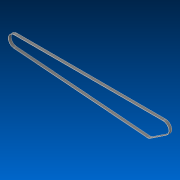
# Autodesk Inventor part: 225T x 9mm Wide Timing Belt (HTD 5mm)(217-3469)
Saved by Autodesk Inventor 2022 (Build 260153000, 153)
## iProperties
Created: 2022-01-07
Part Number: 225T x 9mm Wide Timing Belt (HTD 5mm)(217-3469)
Material: Fiberglass Batt
Document SubType Name: Modeling
Designer: omard
Density: 0.032 g/cm^3
Appearance: Gray
Author: omard
Autodesk Inventor part; units mm, degrees
ref_plane "YZ Plane" through (0, 0, 0) normal (1, 0, 0) x (0, 1, 0)
ref_plane "XZ Plane" through (0, 0, 0) normal (0, 1, 0) x (-1, 0, 0)
ref_plane "XY Plane" through (0, 0, 0) normal (0, 0, 1) x (1, 0, 0)
sketch "Sketch1" plane through (0, 0, 0) normal (0, 0, 1) x (1, 0, 0)
  arc A0 (0, 19.1008) -> (-1.5227, -19.04) centre (0, 0) ccw
  arc A1 (495.3, -19.1008) -> (505.9138, -15.8804) centre (495.3, 0) ccw construction
  line L0 (0, 19.1008) -> (495.3, 19.1008)
  line L1 (495.3, -19.1008) -> (0, -19.1008) construction
  line L2 (495.3, 20.1008) -> (0, 20.1008)
  arc A2 (0, 20.1008) -> (-1.6024, -20.0368) centre (0, 0) ccw
  line L3 (0, -20.1008) -> (495.3, -20.1008) construction
  arc A3 (495.3, -20.1008) -> (500.7083, -19.3595) centre (495.3, 0) ccw construction
  arc A4 (443.6141, -54.6381) -> (450.6749, -52.7999) centre (444.5, -43.561) ccw
  arc A5 (443.5344, -55.635) -> (451.2306, -53.6313) centre (444.5, -43.561) ccw
  line L4 (451.2306, -53.6313) -> (506.4695, -16.7118)
  line L5 (505.9138, -15.8804) -> (450.6749, -52.7999)
  line L6 (443.5344, -55.635) -> (-1.6024, -20.0368)
  line L7 (-1.5227, -19.04) -> (443.6141, -54.6381)
  arc A6 (500.7083, -19.3595) -> (506.4695, -16.7118) centre (495.3, 0) ccw construction
  arc A7 (506.4695, -16.7118) -> (495.3, 20.1008) centre (495.3, 0) ccw
  arc A8 (505.9138, -15.8804) -> (495.3, 19.1008) centre (495.3, 0) ccw
  arc A9 (-1.5227, -19.04) -> (0, -19.1008) centre (0, 0) ccw construction
  arc A10 (-1.6024, -20.0368) -> (0, -20.1008) centre (0, 0) ccw construction
  dimension "d0" = 495.3
  dimension "d1" = 38.2016
  dimension "d2" = 1
  dimension "d5" = 22.225
  dimension "d6" = 50.8
  dimension "d7" = 43.561
  constraints: 25 tangent, 23 point on circle, 16 end point, 11 centre point, 2 coincident, 1 equal radius, 1 horizontal alignment, 1 parallel, 1 point on line
  measures "d0" distance of A1.centre point (0, 0)
  measures "d1" diameter of A1
  measures "d2" distance between parallel lines of L0 L2
  measures "d5" diameter of A4
  measures "d6" horizontal distance of A4.centre A1.centre
  measures "d7" vertical distance of A1.centre A4.centre
extrude "Extrusion1" add sketch "Sketch1" along normal mid plane 9
body "Solid1"
